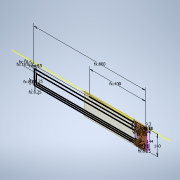
# Autodesk Inventor part: primary_coil_0R2_test_cut
Saved by Autodesk Inventor 2021 (Build 250183000, 183)
## iProperties
Created: 2021-01-20
Part Number: primary_coil_0R2_test_cut
Material: Generic
Document SubType Name: Modeling
Designer: phamv
Density: 1 g/cm^3
Appearance: Default
Author: phamv
Autodesk Inventor part; units mm, degrees
ref_plane "YZ Plane" through (0, 0, 0) normal (1, 0, 0) x (0, 1, 0)
sketch "Sketch1" plane through (0, 0, 0) normal (0, 0, 1) x (1, 0, 0)
  line L0 (-5, -9.3) -> (382, -9.3)
  line L1 (400, -27.3) -> (400, -122)
  line L2 (382, -140) -> (-400, -140)
  line L3 (-400, -140) -> (-400, -32.4)
  line L4 (-5, -9.3) -> (-5, -13.8)
  line L5 (-5, -13.8) -> (380.5, -13.8)
  line L6 (395.5, -28.8) -> (395.5, -120.5)
  line L7 (380.5, -135.5) -> (-395.5, -135.5)
  line L8 (-400, -32.4) -> (369.25, -32.4)
  line L9 (387.25, -50.4) -> (387.25, -109.25)
  line L10 (369.25, -127.25) -> (-387.25, -127.25)
  line L11 (-395.5, -135.5) -> (-395.5, -36.9)
  line L12 (-395.5, -36.9) -> (367.75, -36.9)
  line L13 (382.75, -51.9) -> (382.75, -107.75)
  line L14 (367.75, -122.75) -> (-382.75, -122.75)
  line L15 (-382.75, -122.75) -> (-382.75, -60)
  line L16 (-387.25, -127.25) -> (-387.25, -55.5)
  line L17 (-387.25, -55.5) -> (356.5, -55.5)
  line L18 (374.5, -73.5) -> (374.5, -96.5)
  line L19 (-382.75, -60) -> (355, -60)
  line L20 (370, -75) -> (370, -95)
  line L21 (355, -110) -> (-374.5, -110)
  line L22 (356.5, -114.5) -> (-374.5, -114.5)
  line L23 (-374.5, -114.5) -> (-374.5, -110)
  line L24 (323.0472, -144) -> (407.7972, -144)
  line L25 (407.7972, -144) -> (407.7972, 0)
  line L26 (407.7972, 0) -> (323.0472, 0)
  line L27 (-561.5594, 0) -> (569.3566, 0) projected
  line L28 (323.0472, -65) -> (345.0535, -65)
  line L29 (360.0535, -80) -> (360.0535, -90)
  line L30 (345.0535, -105) -> (323.0472, -105)
  arc A0 (360.0535, -67) -> (358.0535, -65) centre (358.0535, -67) ccw
  arc A1 (360.0535, -80) -> (345.0535, -65) centre (345.0535, -80) ccw
  arc A2 (345.0535, -105) -> (360.0535, -90) centre (345.0535, -90) ccw
  line L31 (323.0472, -18.3) -> (377.5888, -18.3)
  line L32 (377.5888, -18.3) -> (377.5888, -27.9)
  line L33 (377.5888, -27.9) -> (323.0472, -27.9)
  line L34 (323.0472, -41.4) -> (367.1423, -41.4)
  line L35 (367.1423, -41.4) -> (367.1423, -51)
  line L36 (367.1423, -51) -> (323.0472, -51)
  arc A3 (395.5, -28.8) -> (380.5, -13.8) centre (380.5, -28.8) ccw
  arc A4 (382.75, -51.9) -> (367.75, -36.9) centre (367.75, -51.9) ccw
  arc A5 (370, -75) -> (355, -60) centre (355, -75) ccw
  arc A6 (355, -110) -> (370, -95) centre (355, -95) ccw
  arc A7 (367.75, -122.75) -> (382.75, -107.75) centre (367.75, -107.75) ccw
  arc A8 (380.5, -135.5) -> (395.5, -120.5) centre (380.5, -120.5) ccw
  arc A9 (400, -27.3) -> (382, -9.3) centre (382, -27.3) ccw
  arc A10 (387.25, -50.4) -> (369.25, -32.4) centre (369.25, -50.4) ccw
  arc A11 (374.5, -73.5) -> (356.5, -55.5) centre (356.5, -73.5) ccw
  arc A12 (356.5, -114.5) -> (374.5, -96.5) centre (356.5, -96.5) ccw
  arc A13 (369.25, -127.25) -> (387.25, -109.25) centre (369.25, -109.25) ccw
  arc A14 (382, -140) -> (400, -122) centre (382, -122) ccw
  line L37 (323.0472, 0) -> (323.0472, -144)
  point P0 (0, 0)
  point P1 (400, -9.3)
  point P2 (400, -140)
  point P3 (395.5, -13.8)
  point P4 (395.5, -135.5)
  point P5 (387.25, -32.4)
  point P6 (387.25, -127.25)
  point P7 (382.75, -36.9)
  point P8 (382.75, -122.75)
  point P9 (374.5, -55.5)
  point P10 (374.5, -114.5)
  point P11 (370, -60)
  point P12 (370, -110)
  point P13 (0, 0)
  point P14 (400, -9.3)
  point P15 (400, -9.3)
  point P16 (400, -9.3)
  point P17 (395.5, -13.8)
  point P18 (395.5, -13.8)
  point P19 (395.5, -13.8)
  point P20 (387.25, -32.4)
  point P21 (387.25, -32.4)
  point P22 (387.25, -32.4)
  point P23 (382.75, -36.9)
  point P24 (382.75, -36.9)
  point P25 (382.75, -36.9)
  point P26 (374.5, -55.5)
  point P27 (374.5, -55.5)
  point P28 (374.5, -55.5)
  point P29 (370, -60)
  point P30 (370, -60)
  point P31 (370, -60)
  point P32 (370, -110)
  point P33 (370, -110)
  point P34 (370, -110)
  point P35 (374.5, -114.5)
  point P36 (374.5, -114.5)
  point P37 (374.5, -114.5)
  point P38 (382.75, -122.75)
  point P39 (382.75, -122.75)
  point P40 (382.75, -122.75)
  point P41 (387.25, -127.25)
  point P42 (387.25, -127.25)
  point P43 (387.25, -127.25)
  point P44 (395.5, -135.5)
  point P45 (395.5, -135.5)
  point P46 (395.5, -135.5)
  point P47 (400, -140)
  point P48 (400, -140)
  point P49 (400, -140)
  point P50 (360.0535, -65)
  point P51 (360.0535, -105)
  point P52 (323.0472, -13.8)
  point P53 (323.0472, -9.3)
  point P54 (323.0472, -36.9)
  point P55 (323.0472, -32.4)
  point P56 (323.0472, -140)
  point P57 (323.0472, -135.5)
  point P58 (323.0472, -110)
  point P59 (323.0472, -60)
  point P60 (323.0472, -122.75)
  point P61 (323.0472, -114.5)
  point P62 (323.0472, -55.5)
  point P63 (323.0472, -127.25)
  dimension "d91" = 0
  dimension "d1" = 4.5
  dimension "d2" = 4.5
  dimension "d3" = 4.5
  dimension "d5" = 800
  dimension "d6" = 400
  dimension "d7" = 4.5
  dimension "d8" = 4.5
  dimension "d9" = 8.25
  dimension "d10" = 4.5
  dimension "d11" = 18.6
  dimension "d12" = 4.5
  dimension "d13" = 8.25
  dimension "d14" = 4.5
  dimension "d15" = 4.5
  dimension "d16" = 4.5
  dimension "d17" = 8.25
  dimension "d19" = 18.6
  dimension "d20" = 8.25
  dimension "d88" = 4.5
  dimension "d89" = 8.25
  dimension "d90" = 8.25
  dimension "d106" = 144
  dimension "d111" = 5
  dimension "d112" = 5
  dimension "d113" = 2
  dimension "d114" = 15
  dimension "d115" = 4.5
  dimension "d116" = 4.5
  dimension "d117" = 4.5
  dimension "d118" = 4.5
  dimension "d119" = 140
  dimension "d120" = 9.3
  dimension "d121" = 15
  dimension "d122" = 18
  constraints: 74 end point, 54 point on line, 30 point on circle, 30 tangent, 20 horizontal, 19 perpendicular, 15 centre point, 15 vertical, 11 equal radius, 2 parallel, 1 coincident, 1 collinear, 48 other
  measures "d1" distance between parallel lines of L5 L0
  measures "d2" distance between parallel lines of L6 L1
  measures "d3" distance between parallel lines of L2 L7
  measures "d5" distance between parallel lines of L3 L1
  measures "d6" distance from line of point (0, 0) L1
  measures "d7" distance between parallel lines of L3 L11
  measures "d8" distance between parallel lines of L13 L9
  measures "d9" distance between parallel lines of L9 L6
  measures "d10" distance between parallel lines of L8 L12
  measures "d11" distance between parallel lines of L8 L5
  measures "d12" distance between parallel lines of L10 L14
  measures "d13" distance between parallel lines of L7 L10
  measures "d14" distance between parallel lines of L16 L15
  measures "d15" distance between parallel lines of L17 L19
  measures "d16" distance between parallel lines of L20 L18
  measures "d17" distance between parallel lines of L18 L13
  measures "d19" distance between parallel lines of L17 L12
  measures "d20" distance between parallel lines of L11 L16
  measures "d88" distance between parallel lines of L22 L21
  measures "d89" distance between parallel lines of L14 L22
  measures "d90" distance between parallel lines of L15 L23
  measures "d106" distance between parallel lines of L24 L26
  measures "d111" distance between parallel lines of L19 L28
  measures "d112" distance between parallel lines of L21 L30
  measures "d113" radius of A0
  measures "d114" radius of A1
  measures "d115" distance between parallel lines of L5 L31
  measures "d116" distance between parallel lines of L8 L33
  measures "d117" distance between parallel lines of L12 L34
  measures "d118" distance between parallel lines of L17 L36
  measures "d119" distance between parallel lines of L2 L27
  measures "d120" distance between parallel lines of L27 L0
  measures "d121" radius of A3
  measures "d122" radius of A9
extrude "Extrusion1" add sketch "Sketch1" along normal blind 4.5 contours L37 L26 L25 L24 L2 A14 L1 A9 L0 | L5 A3 L6 A8 L7 L37 L10 A13 L9 A10 L8 L33 L32 L31 | L12 A4 L13 A7 L14 L37 L22 A12 L18 A11 L17 L36 L35 L34 | L19 A5 L20 A6 L21 L37 L30 A2 L29 A1 L28
extrude "Extrusion7" add sketch "Sketch1" against normal blind 0.45 contours L37 L26 L25 L24 L2 A14 L1 A9 L0 | L0 A9 L1 A14 L2 L37 L7 A8 L6 A3 L5 | L5 A3 L6 A8 L7 L37 L10 A13 L9 A10 L8 L33 L32 L31 | L31 L32 L33 L37 | L8 A10 L9 A13 L10 L37 L14 A7 L13 A4 L12 | L12 A4 L13 A7 L14 L37 L22 A12 L18 A11 L17 L36 L35 L34 | L34 L35 L36 L37 | L17 A11 L18 A12 L22 L37 L21 A6 L20 A5 L19 | L19 A5 L20 A6 L21 L37 L30 A2 L29 A1 L28 | L28 A1 L29 A2 L30 L37
equation "\"d1\" = wire_diameter"
equation "\"d2\" = wire_diameter"
equation "\"d3\" = wire_diameter"
equation "\"d5\" = track_length"
equation "\"d6\" = 0.5 * track_length"
equation "\"d7\" = wire_diameter"
equation "\"d8\" = wire_diameter"
equation "\"d9\" = distance_between_wires_edge"
equation "\"d10\" = wire_diameter"
equation "\"d11\" = distance_between_wires"
equation "\"d12\" = wire_diameter"
equation "\"d13\" = distance_between_wires_edge"
equation "\"d14\" = wire_diameter"
equation "\"d15\" = wire_diameter"
equation "\"d16\" = wire_diameter"
equation "\"d17\" = distance_between_wires_edge"
equation "\"d19\" = distance_between_wires"
equation "\"d20\" = distance_between_wires_edge"
equation "\"d22\" = wire_diameter"
equation "\"track_length\" = 800"
equation "\"wire_diameter\" = 4.5"
equation "\"distance_between_wires\" = -1.2 * wire_diameter + 0.2 * parameter_6"
equation "\"distance_between_wires_edge\" = 8.25"
equation "\"bend_radius\" = 15"
equation "\"bend_radius_outer\" = 18"
equation "\"parameter_6\" = 120"
body "Solid1"
